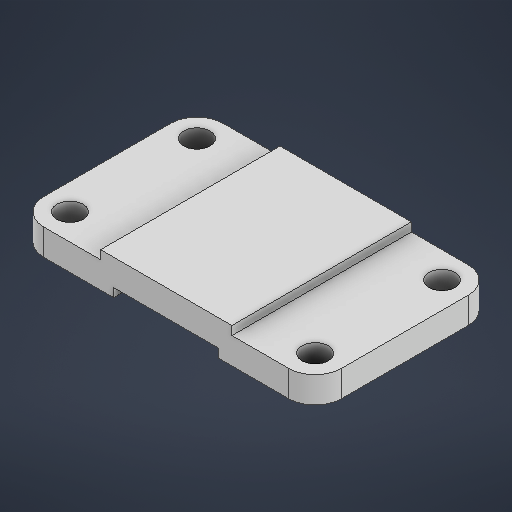
# Autodesk Inventor part: Part4
Saved by Autodesk Inventor 2026 (Build 300175000, 175)
## iProperties
Created: 2025-05-07
Part Number: Part4
Material: Generic
Document SubType Name: Modeling
Designer: Ritul Kumari
Density: 1 g/cm^3
Appearance: Default
Author: Ritul Kumari
Autodesk Inventor part; units mm, degrees
ref_plane "YZ Plane" through (0, 0, 0) normal (1, 0, 0) x (0, 1, 0)
ref_plane "XZ Plane" through (0, 0, 0) normal (0, 1, 0) x (-1, 0, 0)
ref_plane "XY Plane" through (0, 0, 0) normal (0, 0, 1) x (1, 0, 0)
sketch "Sketch1" plane through (0, 0, 0) normal (0, 0, 1) x (1, 0, 0)
  line L0 (-1375.363, 0) -> (-257.763, 0)
  line L1 (-257.763, 0) -> (-257.763, 101.6)
  line L2 (-257.763, 101.6) -> (961.437, 101.6)
  line L3 (961.437, 101.6) -> (961.437, 0)
  line L4 (961.437, 0) -> (2079.037, 0)
  line L5 (2079.037, 0) -> (2079.037, 304.8)
  line L6 (2079.037, 304.8) -> (1113.837, 304.8)
  line L7 (1113.837, 304.8) -> (1113.837, 406.4)
  line L8 (1113.837, 406.4) -> (-410.163, 406.4)
  line L9 (-410.163, 406.4) -> (-410.163, 304.8)
  line L10 (-410.163, 304.8) -> (-1375.363, 304.8)
  line L11 (-1375.363, 304.8) -> (-1375.363, 0)
  point P0 (0, 0)
  dimension "d0" = 1117.6
  dimension "d1" = 101.6
  dimension "d2" = 1219.2
  dimension "d3" = 1117.6
  dimension "d4" = 304.8
  dimension "d5" = 965.2
  dimension "d6" = 1524
  dimension "d7" = 101.6
  constraints: 24 end point, 9 perpendicular, 4 point on line, 1 horizontal
  measures "d0" distance of L0.start L0.end
  measures "d1" distance of L0.end L1.end
  measures "d2" distance of L1.end L2.end
  measures "d3" distance of L3.end L4.end
  measures "d4" distance of L4.end L5.end
  measures "d5" distance of L5.end L6.end
  measures "d6" distance of L7.end L8.end
  measures "d7" distance of L8.end L9.end
extrude "Extrusion1" add sketch "Sketch1" against normal blind 2082.8
fillet "Fillet1" radius 304.8 4 edges at (-1375.363, 152.4, 0) (2079.037, 152.4, 0) (2079.037, 152.4, -2082.8) (-1375.363, 152.4, -2082.8)
sketch "Sketch2" plane through (-410.163, 304.8, 0) normal (0, 1, 0) x (1, 0, 0)
  arc A0 (-660.4, 2082.8) -> (-965.2, 1778) centre (-660.4, 1778) ccw projected
  circle A1 centre (-660.4, 1778) radius 152.4
  arc A2 (-965.2, 304.8) -> (-660.4, 0) centre (-660.4, 304.8) ccw projected
  circle A3 centre (-660.4, 304.8) radius 152.4
  arc A4 (2489.2, 1778) -> (2184.4, 2082.8) centre (2184.4, 1778) ccw projected
  circle A5 centre (2184.4, 1778) radius 152.4
  arc A6 (2184.4, 0) -> (2489.2, 304.8) centre (2184.4, 304.8) ccw projected
  circle A7 centre (2184.4, 304.8) radius 152.4
  point P0 (410.163, 0)
  dimension "d11" = 304.8
  dimension "d12" = 304.8
  dimension "d13" = 304.8
  dimension "d14" = 304.8
  constraints: 5 coincident, 4 centre point
  measures "d11" diameter of A1
  measures "d12" diameter of A3
  measures "d13" diameter of A5
  measures "d14" diameter of A7
hole "Hole1" at (-1070.563, 304.8, -1778) direction (0, -1, 0) diameter 304.8 end through all
sketch "Sketch3" plane through (-410.163, 304.8, 0) normal (0, 1, 0) x (1, 0, 0)
  arc A0 (-965.2, 304.8) -> (-660.4, 0) centre (-660.4, 304.8) ccw projected
  circle A1 centre (-660.4, 304.8) radius 152.4
  point P0 (410.163, 0)
  dimension "d22" = 304.8
  constraints: 1 centre point, 1 coincident
  measures "d22" diameter of A1
hole "Hole2" at (-1070.563, 304.8, -304.8) direction (0, -1, 0) diameter 304.8 end through all
sketch "Sketch4" plane through (1113.837, 304.8, 0) normal (0, 1, 0) x (1, 0, 0)
  arc A0 (965.2, 1778) -> (660.4, 2082.8) centre (660.4, 1778) ccw projected
  circle A1 centre (660.4, 1778) radius 152.4
  point P0 (-1113.837, 0)
  dimension "d30" = 304.8
  constraints: 1 centre point, 1 coincident
  measures "d30" diameter of A1
hole "Hole3" at (1774.237, 304.8, -1778) direction (0, -1, 0) diameter 304.8 end through all
sketch "Sketch5" plane through (1113.837, 304.8, 0) normal (0, 1, 0) x (1, 0, 0)
  arc A0 (660.4, 0) -> (965.2, 304.8) centre (660.4, 304.8) ccw projected
  circle A1 centre (660.4, 304.8) radius 152.4
  point P0 (-1113.837, 0)
  dimension "d38" = 304.8
  constraints: 1 centre point, 1 coincident
  measures "d38" diameter of A1
hole "Hole4" at (1774.237, 304.8, -304.8) direction (0, -1, 0) diameter 304.8 end through all
thread "Thread1" size "M310x6" class "6H" standard "ANSI Metric M Profile" full length
body "Solid1"
